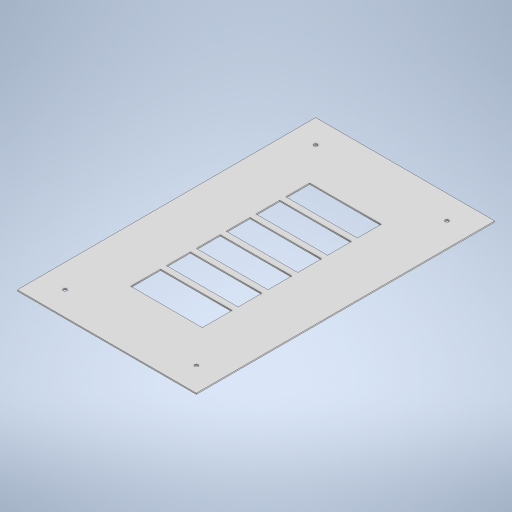
# Autodesk Inventor part: tapa
Saved by Autodesk Inventor 2024 (Build 280153000, 153)
## iProperties
Created: 2023-10-22
Part Number: tapa
Material: Genérico
Document SubType Name: Modeling
Designer: jhonc
Density: 1 g/cm^3
Appearance: Valor por defecto
Author: jhonc
Autodesk Inventor part; units mm, degrees
ref_plane "YZ Plane" through (0, 0, 0) normal (1, 0, 0) x (0, 1, 0)
ref_plane "XZ Plane" through (0, 0, 0) normal (0, 1, 0) x (-1, 0, 0)
ref_plane "XY Plane" through (0, 0, 0) normal (0, 0, 1) x (1, 0, 0)
sketch "Boceto1" plane through (0, 0, 0) normal (0, 1, 0) x (-1, 0, 0)
  line L0 (64.5434, 117.8226) -> (-65.4566, 117.8226)
  line L1 (-65.4566, 117.8226) -> (64.5434, 117.8226)
  line L2 (64.5434, 117.8226) -> (64.5434, -112.1774)
  line L3 (64.5434, -112.1774) -> (-65.4566, -112.1774)
  line L4 (-65.4566, -112.1774) -> (-65.4566, 117.8226)
  circle A0 centre (-55.4566, 107.8226) radius 1.5
  circle A1 centre (-55.4566, 107.8226) radius 1.5
  circle A2 centre (-55.4566, -102.1774) radius 1.5
  circle A3 centre (-55.4566, -102.1774) radius 1.5
  circle A4 centre (54.5563, -102.1774) radius 1.5001
  circle A5 centre (54.5563, 107.8226) radius 1.4926
  line L5 (74.5434, -122.1774) -> (74.5434, 127.8226)
  line L6 (74.5434, 127.8226) -> (-75.4566, 127.8226)
  line L7 (-75.4566, 127.8226) -> (-75.4566, -122.1774)
  line L8 (-75.4566, -122.1774) -> (74.5434, -122.1774)
  line L9 (29.5434, 77.8226) -> (-30.4566, 77.8226)
  line L10 (-30.4566, 77.8226) -> (-30.4566, -82.1774)
  line L11 (29.5434, -82.1774) -> (29.5434, 77.8226)
  line L12 (29.5434, 52.8226) -> (-30.4566, 52.8226)
  line L13 (29.5434, 47.8226) -> (-30.4566, 47.8226)
  line L14 (29.5434, 22.8226) -> (-30.4566, 22.8226)
  line L15 (29.5434, 27.8226) -> (-30.4566, 27.8226)
  line L16 (29.5434, -2.1774) -> (-30.4566, -2.1774)
  line L17 (29.5434, 2.8226) -> (-30.4566, 2.8226)
  line L18 (29.5434, -27.1774) -> (-30.4566, -27.1774)
  line L19 (29.5434, -22.1774) -> (-30.4566, -22.1774)
  line L20 (29.5434, -52.1774) -> (-30.4566, -52.1774)
  line L21 (29.5434, -47.1774) -> (-30.4566, -47.1774)
  line L22 (29.5434, -77.1774) -> (-30.4566, -77.1774)
  line L23 (29.5434, -72.1774) -> (-30.4566, -72.1774)
  point P0 (0, 0)
  dimension "d0" = 10
  dimension "d1" = 60
  dimension "d2" = 160
  dimension "d3" = 45
  dimension "d6" = 50
  dimension "d7" = 25
  dimension "d8" = 5
  dimension "d11" = 25
  constraints: 48 end point, 6 centre point, 5 parallel, 5 perpendicular, 4 point on line, 2 coincident, 2 horizontal, 1 vertical, 33 other
  measures "d0" distance between parallel lines of L2 L5
  measures "d1" distance of L10.end L11.start
  measures "d2" distance of L9.end L10.end
  measures "d3" distance between parallel lines of L7 L10
  measures "d6" distance between parallel lines of L6 L9
  measures "d7" distance between parallel lines of L12 L9
  measures "d8" distance between parallel lines of L13 L12
  measures "d11" distance of L13.start L14.start
extrude "Extrusión1" add sketch "Boceto1" along normal blind 1 contours L2 L3 L4 L0 | L8 L7 L6 L5 | L11 L13 L10 L12 | L11 L14 L10 L15 | L11 L16 L10 L17 | L11 L18 L10 L19 | L11 L20 L10 L21 | L11 L22 L10 L23
